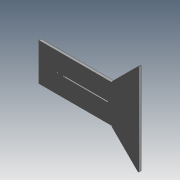
# Autodesk Inventor part: sideplate
Saved by Autodesk Inventor 2015 (Build 190159000, 159)
## iProperties
Created: 2014-08-31
Part Number: sideplate
Material: Generic
Document SubType Name: Modeling
Designer: shohei
Density: 1 g/cm^3
Appearance: Default
Mass: 5703.68 g
Surface Area: 6418.8 cm^2
Volume: 5703.68 cm^3
Author: shohei
Autodesk Inventor part; units mm, degrees
ref_plane "YZ Plane" through (0, 0, 0) normal (1, 0, 0) x (0, 1, 0)
ref_plane "XZ Plane" through (0, 0, 0) normal (0, 1, 0) x (-1, 0, 0)
ref_plane "XY Plane" through (0, 0, 0) normal (0, 0, 1) x (1, 0, 0)
sketch "Sketch1" plane through (0, 0, 0) normal (0, 1, 0) x (-1, 0, 0)
  line L0 (215, 0) -> (800, 0)
  line L1 (800, 0) -> (800, 300)
  line L2 (800, 300) -> (215, 300)
  line L3 (0, 300) -> (0, 0)
  line L4 (-160, 0) -> (960, 0) projected
  line L5 (0, -362.4769) -> (0, 662.4769) projected
  line L6 (960, 0) -> (-160, 0) projected
  arc A0 (10.6069, 510.6063) -> (0, 515) centre (0, 500) ccw
  arc A1 (0, -215) -> (10.6069, -210.6063) centre (0, -200) ccw
  arc A2 (215, 300) -> (210.2772, 310.9261) centre (200, 300) ccw
  arc A3 (210.2772, -10.9261) -> (215, 0) centre (200, 0) ccw
  line L7 (210.2772, 310.9261) -> (10.6069, 510.6063)
  line L8 (210.2772, -10.9261) -> (10.6069, -210.6063)
  line L9 (0, 515) -> (0, 300)
  line L10 (0, -215) -> (0, 0)
  arc A4 (599.9852, 145) -> (604.9434, 150.7503) centre (600, 150) ccw
  circle A5 centre (650, 150) radius 5
  arc A6 (599.9852, 145) -> (599.655, 154.9881) centre (600, 150) ccw
  line L11 (599.9852, 145) -> (600.0264, 145.0001)
  arc A7 (599.9852, 145) -> (599.655, 154.9881) centre (600, 150) ccw
  arc A8 (250.345, 154.9881) -> (250, 145) centre (250, 150) ccw
  line L12 (600.345, 154.9881) -> (250, 154.9881)
  line L13 (599.9852, 145) -> (250, 145)
  point P0 (366.8557, 145.6602)
  point P1 (595.0566, 150.7503)
  dimension "d25" = 800
  dimension "d26" = 30
  dimension "d27" = 30
  dimension "d28" = 200
  dimension "d29" = 200
  dimension "d30" = 30
  dimension "d31" = 30
  dimension "d32" = 200
  dimension "d33" = 200
  dimension "d35" = 10
  dimension "d36" = 10
  dimension "d39" = 50
  dimension "d42" = 300
  dimension "d43" = 300
  dimension "d44" = 150
  dimension "d46" = 10
  dimension "d47" = 150
  dimension "d48" = 250
  dimension "d49" = 350
  constraints: 22 end point, 22 point on circle, 10 point on line, 9 centre point, 4 collinear, 3 tangent, 2 coincident, 2 horizontal, 2 parallel, 1 concentric, 1 perpendicular
  measures "d25" distance of L1.end L3.start
  measures "d26" diameter of A1
  measures "d27" diameter of A0
  measures "d28" distance from line of A0.centre L2
  measures "d29" distance from line of A1.centre L0
  measures "d30" diameter of A2
  measures "d31" diameter of A3
  measures "d32" distance from line of L5 A2.centre
  measures "d33" distance from line of L3 A3.centre
  measures "d35" diameter of A4
  measures "d36" diameter of A5
  measures "d39" distance of A5.centre A4.centre
  measures "d42" distance of L3.end L3.start
  measures "d43" distance of L0.end L1.end
  measures "d44" distance from line of L0 A4.centre
  measures "d46" diameter of A8
  measures "d47" distance from line of L4 A8.centre
  measures "d48" distance from line of L3 A8.centre
  measures "d49" distance of A8.centre A6.centre
extrude "Extrusion2" add sketch "Sketch1" along normal blind 20 contours L4 L3 L5 A0 L7 A2 L2 L1 L0 | A3 L8 A1 L5 L4 | L12 A6
body "Solid2"
